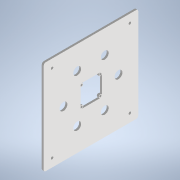
# Autodesk Inventor part: Plate
Saved by Autodesk Inventor 2022 (Build 260153000, 153)
## iProperties
Created: 2022-03-14
Part Number: Plate
Material: Generic
Document SubType Name: Modeling
Designer: ultra
Density: 1 g/cm^3
Appearance: Default
Author: ultra
Autodesk Inventor part; units mm, degrees
ref_plane "YZ Plane" through (0, 0, 0) normal (1, 0, 0) x (0, 1, 0)
ref_plane "XZ Plane" through (0, 0, 0) normal (0, 1, 0) x (-1, 0, 0)
ref_plane "XY Plane" through (0, 0, 0) normal (0, 0, 1) x (1, 0, 0)
sketch "Sketch1" plane through (0, 0, 0) normal (1, 0, 0) x (0, 1, 0)
  line L0 (-76.2, 76.2) -> (76.2, 76.2)
  line L1 (76.2, 76.2) -> (76.2, -76.2)
  line L2 (76.2, -76.2) -> (-76.2, -76.2)
  line L3 (-76.2, -76.2) -> (-76.2, 76.2)
  circle A0 centre (62.8611, 62.86) radius 2.032
  circle A1 centre (-62.8625, -62.8636) radius 2.032
  circle A2 centre (-0.0007, -88.9018) radius 2.032
  circle A3 centre (-62.8625, 62.86) radius 2.032
  circle A4 centre (88.8993, -0.0018) radius 2.032
  circle A5 centre (-88.9007, -0.0018) radius 2.032
  circle A6 centre (62.8611, -62.8636) radius 2.032
  circle A7 centre (-0.0007, 88.8982) radius 2.032
  circle A8 centre (-0.0007, -0.0018) radius 6.35
  dimension "d0" = 152.4
  dimension "d1" = 152.4
  dimension "d5" = 12.7
  constraints: 9 centre point, 8 end point, 2 parallel, 1 horizontal, 1 perpendicular
  measures "d0" distance of L1.end L2.end
  measures "d1" distance of L0.end L1.end
  measures "d5" diameter of A8
extrude "Extrusion2" add sketch "Sketch1" along normal blind 3.175 contours L0 L1 L2 L3 | A8
fillet "Fillet2" radius 3.175 4 edges at (1.5875, 76.2, 76.2) (1.5875, 76.2, -76.2) (1.5875, -76.2, 76.2) (1.5875, -76.2, -76.2)
sketch "Sketch2" plane through (3.175, 0, 0) normal (1, 0, 0) x (0, 0, -1)
  line L0 (-50.8, -50.8) -> (50.8, -50.8)
  line L1 (50.8, -50.8) -> (50.8, 50.8)
  line L2 (50.8, 50.8) -> (-50.8, 50.8)
  line L3 (-50.8, 50.8) -> (-50.8, -50.8)
  line L4 (-50.8, -50.8) -> (50.8, 50.8) construction
  line L5 (50.8, -50.8) -> (-50.8, 50.8) construction
  circle A0 centre (0, 0) radius 12.7
  line L6 (-12.7, 0) -> (-50.8, 38.1)
  line L7 (0, 12.7) -> (-38.1, 50.8)
  line L8 (-38.1, 50.8) -> (0, 12.7)
  line L9 (38.1, 50.8) -> (0, 12.7)
  line L10 (12.7, 0) -> (50.8, 38.1)
  line L11 (12.7, 0) -> (50.8, -38.1)
  line L12 (0, -12.7) -> (38.1, -50.8)
  line L13 (0, -12.7) -> (-38.1, -50.8)
  line L14 (-12.7, 0) -> (-50.8, -38.1)
  dimension "d9" = 101.6
  dimension "d10" = 101.6
  dimension "d11" = 25.4
  constraints: 30 end point, 10 point on line, 5 parallel, 4 point on circle, 2 midpoint, 2 perpendicular, 1 centre point, 1 coincident, 1 collinear, 1 horizontal
  measures "d9" distance of L2.end L1.end
  measures "d10" distance of L1.end L0.end
  measures "d11" diameter of A0
extrude "Extrusion3" [suppressed]
fillet "Fillet3" [suppressed]
sketch "Sketch3" plane through (3.175, 0, 0) normal (1, 0, 0) x (0, 0, -1)
  circle A0 centre (-22.225, -38.4948) radius 6.35
  circle A1 centre (-44.45, 0) radius 6.35
  circle A2 centre (22.225, -38.4948) radius 6.35
  circle A3 centre (-22.225, 38.4948) radius 6.35
  circle A4 centre (22.225, 38.4948) radius 6.35
  circle A5 centre (44.45, 0) radius 6.35
  point P0 (0, 0)
  constraints: 6 centre point
extrude "Extrusion4" cut sketch "Sketch3" against normal blind 25.4
sketch "Sketch4" plane through (3.175, 0, 0) normal (1, 0, 0) x (0, 0, -1)
  arc A0 (17.95, -14.8817) -> (14.6151, -17.9) centre (15.25, -15.25) ccw
  line L0 (17.95, -14.8817) -> (17.95, 14.8817)
  arc A1 (14.6151, 17.9) -> (17.95, 14.8817) centre (15.25, 15.25) ccw
  line L1 (14.6151, 17.9) -> (-14.6151, 17.9)
  arc A2 (-16.7532, 12.9771) -> (-14.6151, 17.9) centre (-15.25, 15.25) ccw
  arc A3 (-16.75, 12.9522) -> (-16.7532, 12.9771) centre (-16.85, 12.9522) ccw
  line L2 (-16.75, 12.9522) -> (-16.75, -12.9522)
  arc A4 (-16.7532, -12.9771) -> (-16.75, -12.9522) centre (-16.85, -12.9522) ccw
  arc A5 (-14.6151, -17.9) -> (-16.7532, -12.9771) centre (-15.25, -15.25) ccw
  line L3 (-14.6151, -17.9) -> (14.6151, -17.9)
  circle A6 centre (-11.1, -15.35) radius 0.6
  circle A7 centre (-11.1, -16.9) radius 0.6
  circle A8 centre (6.4427, -3.2254) radius 0.5
  line L4 (7.15, 15.83) -> (7.15, 17.17)
  arc A9 (7.07, 15.75) -> (7.15, 15.83) centre (7.07, 15.83) ccw
  line L5 (5.73, 15.75) -> (7.07, 15.75)
  arc A10 (5.65, 15.83) -> (5.73, 15.75) centre (5.73, 15.83) ccw
  line L6 (5.65, 17.17) -> (5.65, 15.83)
  arc A11 (5.73, 17.25) -> (5.65, 17.17) centre (5.73, 17.17) ccw
  line L7 (7.07, 17.25) -> (5.73, 17.25)
  arc A12 (7.15, 17.17) -> (7.07, 17.25) centre (7.07, 17.17) ccw
  line L8 (17.3, 4.83) -> (17.3, 6.17)
  arc A13 (17.22, 4.75) -> (17.3, 4.83) centre (17.22, 4.83) ccw
  line L9 (15.88, 4.75) -> (17.22, 4.75)
  arc A14 (15.8, 4.83) -> (15.88, 4.75) centre (15.88, 4.83) ccw
  line L10 (15.8, 6.17) -> (15.8, 4.83)
  arc A15 (15.88, 6.25) -> (15.8, 6.17) centre (15.88, 6.17) ccw
  line L11 (17.22, 6.25) -> (15.88, 6.25)
  arc A16 (17.3, 6.17) -> (17.22, 6.25) centre (17.22, 6.17) ccw
  line L12 (17.2, -10.52) -> (17.2, -9.18)
  arc A17 (17.12, -10.6) -> (17.2, -10.52) centre (17.12, -10.52) ccw
  line L13 (15.78, -10.6) -> (17.12, -10.6)
  arc A18 (15.7, -10.52) -> (15.78, -10.6) centre (15.78, -10.52) ccw
  line L14 (15.7, -9.18) -> (15.7, -10.52)
  arc A19 (15.78, -9.1) -> (15.7, -9.18) centre (15.78, -9.18) ccw
  line L15 (17.12, -9.1) -> (15.78, -9.1)
  arc A20 (17.2, -9.18) -> (17.12, -9.1) centre (17.12, -9.18) ccw
  line L16 (14.45, -7.97) -> (14.45, -6.63)
  arc A21 (14.37, -8.05) -> (14.45, -7.97) centre (14.37, -7.97) ccw
  line L17 (13.03, -8.05) -> (14.37, -8.05)
  arc A22 (12.95, -7.97) -> (13.03, -8.05) centre (13.03, -7.97) ccw
  line L18 (12.95, -6.63) -> (12.95, -7.97)
  arc A23 (13.03, -6.55) -> (12.95, -6.63) centre (13.03, -6.63) ccw
  line L19 (14.37, -6.55) -> (13.03, -6.55)
  arc A24 (14.45, -6.63) -> (14.37, -6.55) centre (14.37, -6.63) ccw
  line L20 (11.7, -11.52) -> (11.7, -10.18)
  arc A25 (11.62, -11.6) -> (11.7, -11.52) centre (11.62, -11.52) ccw
  line L21 (10.28, -11.6) -> (11.62, -11.6)
  arc A26 (10.2, -11.52) -> (10.28, -11.6) centre (10.28, -11.52) ccw
  line L22 (10.2, -10.18) -> (10.2, -11.52)
  arc A27 (10.28, -10.1) -> (10.2, -10.18) centre (10.28, -10.18) ccw
  line L23 (11.62, -10.1) -> (10.28, -10.1)
  arc A28 (11.7, -10.18) -> (11.62, -10.1) centre (11.62, -10.18) ccw
  circle A29 centre (6.25, -16.55) radius 0.75
  circle A30 centre (-12.95, -3.7) radius 0.6
  circle A31 centre (-12.95, -2.2) radius 0.6
  circle A32 centre (-12.95, -0.7) radius 0.6
  circle A33 centre (-15, -2.55) radius 0.5
  line L24 (9.55, -17.22) -> (9.55, -15.88)
  arc A34 (9.47, -17.3) -> (9.55, -17.22) centre (9.47, -17.22) ccw
  line L25 (8.13, -17.3) -> (9.47, -17.3)
  arc A35 (8.05, -17.22) -> (8.13, -17.3) centre (8.13, -17.22) ccw
  line L26 (8.05, -15.88) -> (8.05, -17.22)
  arc A36 (8.13, -15.8) -> (8.05, -15.88) centre (8.13, -15.88) ccw
  line L27 (9.47, -15.8) -> (8.13, -15.8)
  arc A37 (9.55, -15.88) -> (9.47, -15.8) centre (9.47, -15.88) ccw
  line L28 (7.15, 13.11) -> (7.15, 14.45)
  arc A38 (7.07, 13.03) -> (7.15, 13.11) centre (7.07, 13.11) ccw
  line L29 (5.73, 13.03) -> (7.07, 13.03)
  arc A39 (5.65, 13.11) -> (5.73, 13.03) centre (5.73, 13.11) ccw
  line L30 (5.65, 14.45) -> (5.65, 13.11)
  arc A40 (5.73, 14.53) -> (5.65, 14.45) centre (5.73, 14.45) ccw
  line L31 (7.07, 14.53) -> (5.73, 14.53)
  arc A41 (7.15, 14.45) -> (7.07, 14.53) centre (7.07, 14.45) ccw
  line L32 (5.6461, -4.7651) -> (6.9807, -4.7651)
  arc A42 (5.5661, -4.6851) -> (5.6461, -4.7651) centre (5.6461, -4.6851) ccw
  line L33 (5.5661, -4.143) -> (5.5661, -4.6851)
  arc A43 (5.6461, -4.063) -> (5.5661, -4.143) centre (5.6461, -4.143) ccw
  line L34 (6.9807, -4.063) -> (5.6461, -4.063)
  arc A44 (7.0607, -4.143) -> (6.9807, -4.063) centre (6.9807, -4.143) ccw
  line L35 (7.0607, -4.6851) -> (7.0607, -4.143)
  arc A45 (6.9807, -4.7651) -> (7.0607, -4.6851) centre (6.9807, -4.6851) ccw
  line L36 (5.7559, -12.4971) -> (7.4659, -12.4971)
  arc A46 (5.6759, -12.4171) -> (5.7559, -12.4971) centre (5.7559, -12.4171) ccw
  line L37 (5.6759, -11.4299) -> (5.6759, -12.4171)
  arc A47 (5.7559, -11.3499) -> (5.6759, -11.4299) centre (5.7559, -11.4299) ccw
  line L38 (7.4659, -11.3499) -> (5.7559, -11.3499)
  arc A48 (7.5459, -11.4299) -> (7.4659, -11.3499) centre (7.4659, -11.4299) ccw
  line L39 (7.5459, -12.4171) -> (7.5459, -11.4299)
  arc A49 (7.4659, -12.4971) -> (7.5459, -12.4171) centre (7.4659, -12.4171) ccw
  line L40 (-3.7607, -13.1472) -> (-6.2454, -13.1472)
  arc A50 (-3.6107, -13.2972) -> (-3.7607, -13.1472) centre (-3.7607, -13.2972) ccw
  line L41 (-3.6107, -13.9345) -> (-3.6107, -13.2972)
  arc A51 (-3.7607, -14.0845) -> (-3.6107, -13.9345) centre (-3.7607, -13.9345) ccw
  line L42 (-6.2454, -14.0845) -> (-3.7607, -14.0845)
  arc A52 (-6.3954, -13.9345) -> (-6.2454, -14.0845) centre (-6.2454, -13.9345) ccw
  line L43 (-6.3954, -13.2972) -> (-6.3954, -13.9345)
  arc A53 (-6.2454, -13.1472) -> (-6.3954, -13.2972) centre (-6.2454, -13.2972) ccw
  line L44 (-8.6796, 6.7587) -> (-7.8361, 6.7587)
  arc A54 (-8.7596, 6.8387) -> (-8.6796, 6.7587) centre (-8.6796, 6.8387) ccw
  line L45 (-8.7596, 7.1597) -> (-8.7596, 6.8387)
  arc A55 (-8.6796, 7.2397) -> (-8.7596, 7.1597) centre (-8.6796, 7.1597) ccw
  line L46 (-7.8361, 7.2397) -> (-8.6796, 7.2397)
  arc A56 (-7.7561, 7.1597) -> (-7.8361, 7.2397) centre (-7.8361, 7.1597) ccw
  line L47 (-7.7561, 6.8387) -> (-7.7561, 7.1597)
  arc A57 (-7.8361, 6.7587) -> (-7.7561, 6.8387) centre (-7.8361, 6.8387) ccw
  line L48 (-8.7273, 6.0564) -> (-8.7273, 5.7353)
  arc A58 (-8.6473, 6.1364) -> (-8.7273, 6.0564) centre (-8.6473, 6.0564) ccw
  line L49 (-7.8039, 6.1364) -> (-8.6473, 6.1364)
  arc A59 (-7.7239, 6.0564) -> (-7.8039, 6.1364) centre (-7.8039, 6.0564) ccw
  line L50 (-7.7239, 5.7353) -> (-7.7239, 6.0564)
  arc A60 (-7.8039, 5.6553) -> (-7.7239, 5.7353) centre (-7.8039, 5.7353) ccw
  line L51 (-8.6473, 5.6553) -> (-7.8039, 5.6553)
  arc A61 (-8.7273, 5.7353) -> (-8.6473, 5.6553) centre (-8.6473, 5.7353) ccw
  line L52 (-2.4248, 3.855) -> (-2.4248, 3.5921)
  arc A62 (-2.3448, 3.935) -> (-2.4248, 3.855) centre (-2.3448, 3.855) ccw
  line L53 (-1.6366, 3.935) -> (-2.3448, 3.935)
  arc A63 (-1.5566, 3.855) -> (-1.6366, 3.935) centre (-1.6366, 3.855) ccw
  line L54 (-1.5566, 3.5921) -> (-1.5566, 3.855)
  arc A64 (-1.6366, 3.5121) -> (-1.5566, 3.5921) centre (-1.6366, 3.5921) ccw
  line L55 (-2.3448, 3.5121) -> (-1.6366, 3.5121)
  arc A65 (-2.4248, 3.5921) -> (-2.3448, 3.5121) centre (-2.3448, 3.5921) ccw
  line L56 (-2.1101, 10.6062) -> (-2.1101, 10.3433)
  arc A66 (-2.0301, 10.6862) -> (-2.1101, 10.6062) centre (-2.0301, 10.6062) ccw
  line L57 (-1.3218, 10.6862) -> (-2.0301, 10.6862)
  arc A67 (-1.2418, 10.6062) -> (-1.3218, 10.6862) centre (-1.3218, 10.6062) ccw
  line L58 (-1.2418, 10.3433) -> (-1.2418, 10.6062)
  arc A68 (-1.3218, 10.2633) -> (-1.2418, 10.3433) centre (-1.3218, 10.3433) ccw
  line L59 (-2.0301, 10.2633) -> (-1.3218, 10.2633)
  arc A69 (-2.1101, 10.3433) -> (-2.0301, 10.2633) centre (-2.0301, 10.3433) ccw
  line L60 (4.251, 0.1966) -> (4.251, -0.0664)
  arc A70 (4.331, 0.2766) -> (4.251, 0.1966) centre (4.331, 0.1966) ccw
  line L61 (5.0392, 0.2766) -> (4.331, 0.2766)
  arc A71 (5.1192, 0.1966) -> (5.0392, 0.2766) centre (5.0392, 0.1966) ccw
  line L62 (5.1192, -0.0664) -> (5.1192, 0.1966)
  arc A72 (5.0392, -0.1464) -> (5.1192, -0.0664) centre (5.0392, -0.0664) ccw
  line L63 (4.331, -0.1464) -> (5.0392, -0.1464)
  arc A73 (4.251, -0.0664) -> (4.331, -0.1464) centre (4.331, -0.0664) ccw
  line L64 (4.251, -2.0073) -> (4.251, -2.2703)
  arc A74 (4.331, -1.9273) -> (4.251, -2.0073) centre (4.331, -2.0073) ccw
  line L65 (5.0392, -1.9273) -> (4.331, -1.9273)
  arc A75 (5.1192, -2.0073) -> (5.0392, -1.9273) centre (5.0392, -2.0073) ccw
  line L66 (5.1192, -2.2703) -> (5.1192, -2.0073)
  arc A76 (5.0392, -2.3503) -> (5.1192, -2.2703) centre (5.0392, -2.2703) ccw
  line L67 (4.331, -2.3503) -> (5.0392, -2.3503)
  arc A77 (4.251, -2.2703) -> (4.331, -2.3503) centre (4.331, -2.2703) ccw
  line L68 (5.5661, -5.3938) -> (5.5661, -5.6568)
  arc A78 (5.6461, -5.3138) -> (5.5661, -5.3938) centre (5.6461, -5.3938) ccw
  line L69 (6.3543, -5.3138) -> (5.6461, -5.3138)
  arc A79 (6.4343, -5.3938) -> (6.3543, -5.3138) centre (6.3543, -5.3938) ccw
  line L70 (6.4343, -5.6568) -> (6.4343, -5.3938)
  arc A80 (6.3543, -5.7368) -> (6.4343, -5.6568) centre (6.3543, -5.6568) ccw
  line L71 (5.6461, -5.7368) -> (6.3543, -5.7368)
  arc A81 (5.5661, -5.6568) -> (5.6461, -5.7368) centre (5.6461, -5.6568) ccw
  line L72 (5.6014, -10.4773) -> (5.6014, -10.7403)
  arc A82 (5.6814, -10.3973) -> (5.6014, -10.4773) centre (5.6814, -10.4773) ccw
  line L73 (6.3896, -10.3973) -> (5.6814, -10.3973)
  arc A83 (6.4696, -10.4773) -> (6.3896, -10.3973) centre (6.3896, -10.4773) ccw
  line L74 (6.4696, -10.7403) -> (6.4696, -10.4773)
  arc A84 (6.3896, -10.8203) -> (6.4696, -10.7403) centre (6.3896, -10.7403) ccw
  line L75 (5.6814, -10.8203) -> (6.3896, -10.8203)
  arc A85 (5.6014, -10.7403) -> (5.6814, -10.8203) centre (5.6814, -10.7403) ccw
  line L76 (-2.5133, -12.7708) -> (-2.5133, -13.0338)
  arc A86 (-2.4333, -12.6908) -> (-2.5133, -12.7708) centre (-2.4333, -12.7708) ccw
  line L77 (-1.7251, -12.6908) -> (-2.4333, -12.6908)
  arc A87 (-1.6451, -12.7708) -> (-1.7251, -12.6908) centre (-1.7251, -12.7708) ccw
  line L78 (-1.6451, -13.0338) -> (-1.6451, -12.7708)
  arc A88 (-1.7251, -13.1138) -> (-1.6451, -13.0338) centre (-1.7251, -13.0338) ccw
  line L79 (-2.4333, -13.1138) -> (-1.7251, -13.1138)
  arc A89 (-2.5133, -13.0338) -> (-2.4333, -13.1138) centre (-2.4333, -13.0338) ccw
  line L80 (-2.5327, -13.863) -> (-2.5327, -14.1668)
  arc A90 (-2.4527, -13.783) -> (-2.5327, -13.863) centre (-2.4527, -13.863) ccw
  line L81 (-1.6863, -13.783) -> (-2.4527, -13.783)
  arc A91 (-1.6063, -13.863) -> (-1.6863, -13.783) centre (-1.6863, -13.863) ccw
  line L82 (-1.6063, -14.1668) -> (-1.6063, -13.863)
  arc A92 (-1.6863, -14.2468) -> (-1.6063, -14.1668) centre (-1.6863, -14.1668) ccw
  line L83 (-2.4527, -14.2468) -> (-1.6863, -14.2468)
  arc A93 (-2.5327, -14.1668) -> (-2.4527, -14.2468) centre (-2.4527, -14.1668) ccw
  line L84 (-4.2466, 7.147) -> (-3.9765, 7.147)
  arc A94 (-4.3266, 7.227) -> (-4.2466, 7.147) centre (-4.2466, 7.227) ccw
  line L85 (-4.3266, 7.9294) -> (-4.3266, 7.227)
  arc A95 (-4.2466, 8.0094) -> (-4.3266, 7.9294) centre (-4.2466, 7.9294) ccw
  line L86 (-3.9765, 8.0094) -> (-4.2466, 8.0094)
  arc A96 (-3.8965, 7.9294) -> (-3.9765, 8.0094) centre (-3.9765, 7.9294) ccw
  line L87 (-3.8965, 7.227) -> (-3.8965, 7.9294)
  arc A97 (-3.9765, 7.147) -> (-3.8965, 7.227) centre (-3.9765, 7.227) ccw
  line L88 (-4.3762, 4.795) -> (-4.3762, 4.0926)
  arc A98 (-4.2962, 4.875) -> (-4.3762, 4.795) centre (-4.2962, 4.795) ccw
  line L89 (-4.0261, 4.875) -> (-4.2962, 4.875)
  arc A99 (-3.9461, 4.795) -> (-4.0261, 4.875) centre (-4.0261, 4.795) ccw
  line L90 (-3.9461, 4.0926) -> (-3.9461, 4.795)
  arc A100 (-4.0261, 4.0126) -> (-3.9461, 4.0926) centre (-4.0261, 4.0926) ccw
  line L91 (-4.2962, 4.0126) -> (-4.0261, 4.0126)
  arc A101 (-4.3762, 4.0926) -> (-4.2962, 4.0126) centre (-4.2962, 4.0926) ccw
  line L92 (-7.8593, 3.5305) -> (-7.8593, 2.8281)
  arc A102 (-7.7793, 3.6105) -> (-7.8593, 3.5305) centre (-7.7793, 3.5305) ccw
  line L93 (-7.5091, 3.6105) -> (-7.7793, 3.6105)
  arc A103 (-7.4291, 3.5305) -> (-7.5091, 3.6105) centre (-7.5091, 3.5305) ccw
  line L94 (-7.4291, 2.8281) -> (-7.4291, 3.5305)
  arc A104 (-7.5091, 2.7481) -> (-7.4291, 2.8281) centre (-7.5091, 2.8281) ccw
  line L95 (-7.7793, 2.7481) -> (-7.5091, 2.7481)
  arc A105 (-7.8593, 2.8281) -> (-7.7793, 2.7481) centre (-7.7793, 2.8281) ccw
  line L96 (8.2438, -6.8732) -> (8.2438, -7.5756)
  arc A106 (8.3238, -6.7932) -> (8.2438, -6.8732) centre (8.3238, -6.8732) ccw
  line L97 (8.594, -6.7932) -> (8.3238, -6.7932)
  arc A107 (8.674, -6.8732) -> (8.594, -6.7932) centre (8.594, -6.8732) ccw
  line L98 (8.674, -7.5756) -> (8.674, -6.8732)
  arc A108 (8.594, -7.6556) -> (8.674, -7.5756) centre (8.594, -7.5756) ccw
  line L99 (8.3238, -7.6556) -> (8.594, -7.6556)
  arc A109 (8.2438, -7.5756) -> (8.3238, -7.6556) centre (8.3238, -7.5756) ccw
  line L100 (4.0983, -7.1851) -> (4.0983, -7.8875)
  arc A110 (4.1783, -7.1051) -> (4.0983, -7.1851) centre (4.1783, -7.1851) ccw
  line L101 (4.4484, -7.1051) -> (4.1783, -7.1051)
  arc A111 (4.5284, -7.1851) -> (4.4484, -7.1051) centre (4.4484, -7.1851) ccw
  line L102 (4.5284, -7.8875) -> (4.5284, -7.1851)
  arc A112 (4.4484, -7.9675) -> (4.5284, -7.8875) centre (4.4484, -7.8875) ccw
  line L103 (4.1783, -7.9675) -> (4.4484, -7.9675)
  arc A113 (4.0983, -7.8875) -> (4.1783, -7.9675) centre (4.1783, -7.8875) ccw
  line L104 (1.7294, -13.1227) -> (1.7294, -13.8251)
  arc A114 (1.8094, -13.0427) -> (1.7294, -13.1227) centre (1.8094, -13.1227) ccw
  line L105 (2.0795, -13.0427) -> (1.8094, -13.0427)
  arc A115 (2.1595, -13.1227) -> (2.0795, -13.0427) centre (2.0795, -13.1227) ccw
  line L106 (2.1595, -13.8251) -> (2.1595, -13.1227)
  arc A116 (2.0795, -13.9051) -> (2.1595, -13.8251) centre (2.0795, -13.8251) ccw
  line L107 (1.8094, -13.9051) -> (2.0795, -13.9051)
  arc A117 (1.7294, -13.8251) -> (1.8094, -13.9051) centre (1.8094, -13.8251) ccw
  line L108 (0.6373, -13.1227) -> (0.6373, -13.8251)
  arc A118 (0.7173, -13.0427) -> (0.6373, -13.1227) centre (0.7173, -13.1227) ccw
  line L109 (0.9875, -13.0427) -> (0.7173, -13.0427)
  arc A119 (1.0675, -13.1227) -> (0.9875, -13.0427) centre (0.9875, -13.1227) ccw
  line L110 (1.0675, -13.8251) -> (1.0675, -13.1227)
  arc A120 (0.9875, -13.9051) -> (1.0675, -13.8251) centre (0.9875, -13.8251) ccw
  line L111 (0.7173, -13.9051) -> (0.9875, -13.9051)
  arc A121 (0.6373, -13.8251) -> (0.7173, -13.9051) centre (0.7173, -13.8251) ccw
  line L112 (-0.5491, -13.0325) -> (-0.5491, -13.8891)
  arc A122 (-0.4691, -12.9525) -> (-0.5491, -13.0325) centre (-0.4691, -13.0325) ccw
  line L113 (-0.0298, -12.9525) -> (-0.4691, -12.9525)
  arc A123 (0.0502, -13.0325) -> (-0.0298, -12.9525) centre (-0.0298, -13.0325) ccw
  line L114 (0.0502, -13.8891) -> (0.0502, -13.0325)
  arc A124 (-0.0298, -13.9691) -> (0.0502, -13.8891) centre (-0.0298, -13.8891) ccw
  line L115 (-0.4691, -13.9691) -> (-0.0298, -13.9691)
  arc A125 (-0.5491, -13.8891) -> (-0.4691, -13.9691) centre (-0.4691, -13.8891) ccw
  line L116 (-7.6347, -13.1227) -> (-7.6347, -13.8251)
  arc A126 (-7.5547, -13.0427) -> (-7.6347, -13.1227) centre (-7.5547, -13.1227) ccw
  line L117 (-7.2846, -13.0427) -> (-7.5547, -13.0427)
  arc A127 (-7.2046, -13.1227) -> (-7.2846, -13.0427) centre (-7.2846, -13.1227) ccw
  line L118 (-7.2046, -13.8251) -> (-7.2046, -13.1227)
  arc A128 (-7.2846, -13.9051) -> (-7.2046, -13.8251) centre (-7.2846, -13.8251) ccw
  line L119 (-7.5547, -13.9051) -> (-7.2846, -13.9051)
  arc A129 (-7.6347, -13.8251) -> (-7.5547, -13.9051) centre (-7.5547, -13.8251) ccw
  line L120 (-11.5137, -7.8762) -> (-11.5137, -8.5786)
  arc A130 (-11.4337, -7.7962) -> (-11.5137, -7.8762) centre (-11.4337, -7.8762) ccw
  line L121 (-11.1636, -7.7962) -> (-11.4337, -7.7962)
  arc A131 (-11.0836, -7.8762) -> (-11.1636, -7.7962) centre (-11.1636, -7.8762) ccw
  line L122 (-11.0836, -8.5786) -> (-11.0836, -7.8762)
  arc A132 (-11.1636, -8.6586) -> (-11.0836, -8.5786) centre (-11.1636, -8.5786) ccw
  line L123 (-11.4337, -8.6586) -> (-11.1636, -8.6586)
  arc A133 (-11.5137, -8.5786) -> (-11.4337, -8.6586) centre (-11.4337, -8.5786) ccw
  line L124 (-11.5137, -5.7855) -> (-11.5137, -6.4879)
  arc A134 (-11.4337, -5.7055) -> (-11.5137, -5.7855) centre (-11.4337, -5.7855) ccw
  line L125 (-11.1636, -5.7055) -> (-11.4337, -5.7055)
  arc A135 (-11.0836, -5.7855) -> (-11.1636, -5.7055) centre (-11.1636, -5.7855) ccw
  line L126 (-11.0836, -6.4879) -> (-11.0836, -5.7855)
  arc A136 (-11.1636, -6.5679) -> (-11.0836, -6.4879) centre (-11.1636, -6.4879) ccw
  line L127 (-11.4337, -6.5679) -> (-11.1636, -6.5679)
  arc A137 (-11.5137, -6.4879) -> (-11.4337, -6.5679) centre (-11.4337, -6.4879) ccw
  line L128 (-6.8045, 2.6819) -> (-6.3852, 2.6819)
  arc A138 (-6.8845, 2.7619) -> (-6.8045, 2.6819) centre (-6.8045, 2.7619) ccw
  line L129 (-6.8845, 3.604) -> (-6.8845, 2.7619)
  arc A139 (-6.8045, 3.684) -> (-6.8845, 3.604) centre (-6.8045, 3.604) ccw
  line L130 (-6.3852, 3.684) -> (-6.8045, 3.684)
  arc A140 (-6.3052, 3.604) -> (-6.3852, 3.684) centre (-6.3852, 3.604) ccw
  line L131 (-6.3052, 2.7619) -> (-6.3052, 3.604)
  arc A141 (-6.3852, 2.6819) -> (-6.3052, 2.7619) centre (-6.3852, 2.7619) ccw
  line L132 (4.2459, -1.3202) -> (5.1267, -1.3202)
  arc A142 (4.1659, -1.2402) -> (4.2459, -1.3202) centre (4.2459, -1.2402) ccw
  line L133 (4.1659, -0.8183) -> (4.1659, -1.2402)
  arc A143 (4.2459, -0.7383) -> (4.1659, -0.8183) centre (4.2459, -0.8183) ccw
  line L134 (5.1267, -0.7383) -> (4.2459, -0.7383)
  arc A144 (5.2067, -0.8183) -> (5.1267, -0.7383) centre (5.1267, -0.8183) ccw
  line L135 (5.2067, -1.2402) -> (5.2067, -0.8183)
  arc A145 (5.1267, -1.3202) -> (5.2067, -1.2402) centre (5.1267, -1.2402) ccw
  line L136 (8.5655, 12.3987) -> (9.3164, 12.3987)
  arc A146 (8.4855, 12.4787) -> (8.5655, 12.3987) centre (8.5655, 12.4787) ccw
  line L137 (8.4855, 13.8248) -> (8.4855, 12.4787)
  arc A147 (8.5655, 13.9048) -> (8.4855, 13.8248) centre (8.5655, 13.8248) ccw
  line L138 (9.3164, 13.9048) -> (8.5655, 13.9048)
  arc A148 (9.3964, 13.8248) -> (9.3164, 13.9048) centre (9.3164, 13.8248) ccw
  line L139 (9.3964, 12.4787) -> (9.3964, 13.8248)
  arc A149 (9.3164, 12.3987) -> (9.3964, 12.4787) centre (9.3164, 12.4787) ccw
  line L140 (8.5655, 15.1054) -> (9.234, 15.1054)
  arc A150 (8.4855, 15.1854) -> (8.5655, 15.1054) centre (8.5655, 15.1854) ccw
  line L141 (8.4855, 16.6154) -> (8.4855, 15.1854)
  arc A151 (8.5655, 16.6954) -> (8.4855, 16.6154) centre (8.5655, 16.6154) ccw
  line L142 (9.234, 16.6954) -> (8.5655, 16.6954)
  arc A152 (9.314, 16.6154) -> (9.234, 16.6954) centre (9.234, 16.6154) ccw
  line L143 (9.314, 15.1854) -> (9.314, 16.6154)
  arc A153 (9.234, 15.1054) -> (9.314, 15.1854) centre (9.234, 15.1854) ccw
  line L144 (3.1491, 10.119) -> (3.4442, 10.119)
  arc A154 (3.0691, 10.199) -> (3.1491, 10.119) centre (3.1491, 10.199) ccw
  line L145 (3.0691, 10.9694) -> (3.0691, 10.199)
  arc A155 (3.1491, 11.0494) -> (3.0691, 10.9694) centre (3.1491, 10.9694) ccw
  line L146 (3.4442, 11.0494) -> (3.1491, 11.0494)
  arc A156 (3.5242, 10.9694) -> (3.4442, 11.0494) centre (3.4442, 10.9694) ccw
  line L147 (3.5242, 10.199) -> (3.5242, 10.9694)
  arc A157 (3.4442, 10.119) -> (3.5242, 10.199) centre (3.4442, 10.199) ccw
  line L148 (4.1659, 10.941) -> (4.1659, 10.1706)
  arc A158 (4.2459, 11.021) -> (4.1659, 10.941) centre (4.2459, 10.941) ccw
  line L149 (4.5409, 11.021) -> (4.2459, 11.021)
  arc A159 (4.6209, 10.941) -> (4.5409, 11.021) centre (4.5409, 10.941) ccw
  line L150 (4.6209, 10.1706) -> (4.6209, 10.941)
  arc A160 (4.5409, 10.0906) -> (4.6209, 10.1706) centre (4.5409, 10.1706) ccw
  line L151 (4.2459, 10.0906) -> (4.5409, 10.0906)
  arc A161 (4.1659, 10.1706) -> (4.2459, 10.0906) centre (4.2459, 10.1706) ccw
  line L152 (5.2631, 10.941) -> (5.2631, 10.1706)
  arc A162 (5.3431, 11.021) -> (5.2631, 10.941) centre (5.3431, 10.941) ccw
  line L153 (5.6381, 11.021) -> (5.3431, 11.021)
  arc A163 (5.7181, 10.941) -> (5.6381, 11.021) centre (5.6381, 10.941) ccw
  line L154 (5.7181, 10.1706) -> (5.7181, 10.941)
  arc A164 (5.6381, 10.0906) -> (5.7181, 10.1706) centre (5.6381, 10.1706) ccw
  line L155 (5.3431, 10.0906) -> (5.6381, 10.0906)
  arc A165 (5.2631, 10.1706) -> (5.3431, 10.0906) centre (5.3431, 10.1706) ccw
  line L156 (6.7177, 10.941) -> (6.7177, 10.1706)
  arc A166 (6.7977, 11.021) -> (6.7177, 10.941) centre (6.7977, 10.941) ccw
  line L157 (7.0927, 11.021) -> (6.7977, 11.021)
  arc A167 (7.1727, 10.941) -> (7.0927, 11.021) centre (7.0927, 10.941) ccw
  line L158 (7.1727, 10.1706) -> (7.1727, 10.941)
  arc A168 (7.0927, 10.0906) -> (7.1727, 10.1706) centre (7.0927, 10.1706) ccw
  line L159 (6.7977, 10.0906) -> (7.0927, 10.0906)
  arc A169 (6.7177, 10.1706) -> (6.7977, 10.0906) centre (6.7977, 10.1706) ccw
  line L160 (7.7678, 10.895) -> (7.7678, 10.1246)
  arc A170 (7.8478, 10.975) -> (7.7678, 10.895) centre (7.8478, 10.895) ccw
  line L161 (8.1429, 10.975) -> (7.8478, 10.975)
  arc A171 (8.2229, 10.895) -> (8.1429, 10.975) centre (8.1429, 10.895) ccw
  line L162 (8.2229, 10.1246) -> (8.2229, 10.895)
  arc A172 (8.1429, 10.0446) -> (8.2229, 10.1246) centre (8.1429, 10.1246) ccw
  line L163 (7.8478, 10.0446) -> (8.1429, 10.0446)
  arc A173 (7.7678, 10.1246) -> (7.8478, 10.0446) centre (7.8478, 10.1246) ccw
  line L164 (4.1659, 8.6981) -> (4.1659, 7.9277)
  arc A174 (4.2459, 8.7781) -> (4.1659, 8.6981) centre (4.2459, 8.6981) ccw
  line L165 (4.5409, 8.7781) -> (4.2459, 8.7781)
  arc A175 (4.6209, 8.6981) -> (4.5409, 8.7781) centre (4.5409, 8.6981) ccw
  line L166 (4.6209, 7.9277) -> (4.6209, 8.6981)
  arc A176 (4.5409, 7.8477) -> (4.6209, 7.9277) centre (4.5409, 7.9277) ccw
  line L167 (4.2459, 7.8477) -> (4.5409, 7.8477)
  arc A177 (4.1659, 7.9277) -> (4.2459, 7.8477) centre (4.2459, 7.9277) ccw
  line L168 (4.1422, 6.6231) -> (4.1422, 5.8527)
  arc A178 (4.2222, 6.7031) -> (4.1422, 6.6231) centre (4.2222, 6.6231) ccw
  line L169 (4.5172, 6.7031) -> (4.2222, 6.7031)
  arc A179 (4.5972, 6.6231) -> (4.5172, 6.7031) centre (4.5172, 6.6231) ccw
  line L170 (4.5972, 5.8527) -> (4.5972, 6.6231)
  arc A180 (4.5172, 5.7727) -> (4.5972, 5.8527) centre (4.5172, 5.8527) ccw
  line L171 (4.2222, 5.7727) -> (4.5172, 5.7727)
  arc A181 (4.1422, 5.8527) -> (4.2222, 5.7727) centre (4.2222, 5.8527) ccw
  line L172 (4.331, -14.4484) -> (5.6381, -14.4484)
  arc A182 (4.251, -14.3684) -> (4.331, -14.4484) centre (4.331, -14.3684) ccw
  line L173 (4.251, -13.7408) -> (4.251, -14.3684)
  arc A183 (4.331, -13.6608) -> (4.251, -13.7408) centre (4.331, -13.7408) ccw
  line L174 (5.6381, -13.6608) -> (4.331, -13.6608)
  arc A184 (5.7181, -13.7408) -> (5.6381, -13.6608) centre (5.6381, -13.7408) ccw
  line L175 (5.7181, -14.3684) -> (5.7181, -13.7408)
  arc A185 (5.6381, -14.4484) -> (5.7181, -14.3684) centre (5.6381, -14.3684) ccw
  line L176 (7.0497, -14.4484) -> (8.471, -14.4484)
  arc A186 (6.9697, -14.3684) -> (7.0497, -14.4484) centre (7.0497, -14.3684) ccw
  line L177 (6.9697, -13.7408) -> (6.9697, -14.3684)
  arc A187 (7.0497, -13.6608) -> (6.9697, -13.7408) centre (7.0497, -13.7408) ccw
  line L178 (8.471, -13.6608) -> (7.0497, -13.6608)
  arc A188 (8.551, -13.7408) -> (8.471, -13.6608) centre (8.471, -13.7408) ccw
  line L179 (8.551, -14.3684) -> (8.551, -13.7408)
  arc A189 (8.471, -14.4484) -> (8.551, -14.3684) centre (8.471, -14.3684) ccw
  line L180 (16.0437, 3.0276) -> (16.0437, 3.4967)
  line L181 (16.7651, 3.0276) -> (16.0437, 3.0276)
  arc A190 (16.9393, 2.8534) -> (16.7651, 3.0276) centre (16.7651, 2.8534) ccw
  line L182 (16.9393, 2.6792) -> (16.9393, 2.8534)
  arc A191 (16.7651, 2.505) -> (16.9393, 2.6792) centre (16.7651, 2.6792) ccw
  line L183 (16.0437, 2.505) -> (16.7651, 2.505)
  line L184 (16.0437, 1.7552) -> (16.0437, 2.505)
  line L185 (16.7651, 1.7552) -> (16.0437, 1.7552)
  arc A192 (16.9393, 1.581) -> (16.7651, 1.7552) centre (16.7651, 1.581) ccw
  line L186 (16.9393, 1.4068) -> (16.9393, 1.581)
  arc A193 (16.7651, 1.2326) -> (16.9393, 1.4068) centre (16.7651, 1.4068) ccw
  line L187 (16.0437, 1.2326) -> (16.7651, 1.2326)
  line L188 (16.0437, 0.4828) -> (16.0437, 1.2326)
  line L189 (16.7651, 0.4828) -> (16.0437, 0.4828)
  arc A194 (16.9393, 0.3086) -> (16.7651, 0.4828) centre (16.7651, 0.3086) ccw
  line L190 (16.9393, 0.1344) -> (16.9393, 0.3086)
  arc A195 (16.7651, -0.0398) -> (16.9393, 0.1344) centre (16.7651, 0.1344) ccw
  line L191 (16.0437, -0.0398) -> (16.7651, -0.0398)
  line L192 (16.0437, -0.7897) -> (16.0437, -0.0398)
  line L193 (16.7651, -0.7897) -> (16.0437, -0.7897)
  arc A196 (16.9393, -0.9638) -> (16.7651, -0.7897) centre (16.7651, -0.9638) ccw
  line L194 (16.9393, -1.138) -> (16.9393, -0.9638)
  arc A197 (16.7651, -1.3122) -> (16.9393, -1.138) centre (16.7651, -1.138) ccw
  line L195 (16.0437, -1.3122) -> (16.7651, -1.3122)
  line L196 (16.0437, -2.0621) -> (16.0437, -1.3122)
  line L197 (16.7651, -2.0621) -> (16.0437, -2.0621)
  arc A198 (16.9393, -2.2362) -> (16.7651, -2.0621) centre (16.7651, -2.2362) ccw
  line L198 (16.9393, -2.4104) -> (16.9393, -2.2362)
  arc A199 (16.7651, -2.5846) -> (16.9393, -2.4104) centre (16.7651, -2.4104) ccw
  line L199 (16.0437, -2.5846) -> (16.7651, -2.5846)
  line L200 (16.0437, -3.2742) -> (16.0437, -2.5846)
  line L201 (13.0463, -3.2742) -> (16.0437, -3.2742)
  line L202 (13.0463, -2.5846) -> (13.0463, -3.2742)
  line L203 (12.3249, -2.5846) -> (13.0463, -2.5846)
  arc A200 (12.1507, -2.4104) -> (12.3249, -2.5846) centre (12.3249, -2.4104) ccw
  line L204 (12.1507, -2.2362) -> (12.1507, -2.4104)
  arc A201 (12.3249, -2.0621) -> (12.1507, -2.2362) centre (12.3249, -2.2362) ccw
  line L205 (13.0463, -2.0621) -> (12.3249, -2.0621)
  line L206 (13.0463, -1.3122) -> (13.0463, -2.0621)
  line L207 (12.3249, -1.3122) -> (13.0463, -1.3122)
  arc A202 (12.1507, -1.138) -> (12.3249, -1.3122) centre (12.3249, -1.138) ccw
  line L208 (12.1507, -0.9638) -> (12.1507, -1.138)
  arc A203 (12.3249, -0.7897) -> (12.1507, -0.9638) centre (12.3249, -0.9638) ccw
  line L209 (13.0463, -0.7897) -> (12.3249, -0.7897)
  line L210 (13.0463, -0.0398) -> (13.0463, -0.7897)
  line L211 (12.3249, -0.0398) -> (13.0463, -0.0398)
  arc A204 (12.1507, 0.1344) -> (12.3249, -0.0398) centre (12.3249, 0.1344) ccw
  line L212 (12.1507, 0.3086) -> (12.1507, 0.1344)
  arc A205 (12.3249, 0.4828) -> (12.1507, 0.3086) centre (12.3249, 0.3086) ccw
  line L213 (13.0463, 0.4828) -> (12.3249, 0.4828)
  line L214 (13.0463, 1.2326) -> (13.0463, 0.4828)
  line L215 (12.3249, 1.2326) -> (13.0463, 1.2326)
  arc A206 (12.1507, 1.4068) -> (12.3249, 1.2326) centre (12.3249, 1.4068) ccw
  line L216 (12.1507, 1.581) -> (12.1507, 1.4068)
  arc A207 (12.3249, 1.7552) -> (12.1507, 1.581) centre (12.3249, 1.581) ccw
  line L217 (13.0463, 1.7552) -> (12.3249, 1.7552)
  line L218 (13.0463, 2.505) -> (13.0463, 1.7552)
  line L219 (12.3249, 2.505) -> (13.0463, 2.505)
  arc A208 (12.1507, 2.6792) -> (12.3249, 2.505) centre (12.3249, 2.6792) ccw
  line L220 (12.1507, 2.8534) -> (12.1507, 2.6792)
  arc A209 (12.3249, 3.0276) -> (12.1507, 2.8534) centre (12.3249, 2.8534) ccw
  line L221 (13.0463, 3.0276) -> (12.3249, 3.0276)
  line L222 (13.0463, 3.4967) -> (13.0463, 3.0276)
  line L223 (16.0437, 3.4967) -> (13.0463, 3.4967)
  line L224 (5.0276, -8.661) -> (7.7758, -8.661)
  arc A210 (4.9476, -8.581) -> (5.0276, -8.661) centre (5.0276, -8.581) ccw
  line L225 (4.9476, -7.1347) -> (4.9476, -8.581)
  arc A211 (5.0276, -7.0547) -> (4.9476, -7.1347) centre (5.0276, -7.1347) ccw
  line L226 (7.7758, -7.0547) -> (5.0276, -7.0547)
  arc A212 (7.8558, -7.1347) -> (7.7758, -7.0547) centre (7.7758, -7.1347) ccw
  line L227 (7.8558, -8.581) -> (7.8558, -7.1347)
  arc A213 (7.7758, -8.661) -> (7.8558, -8.581) centre (7.7758, -8.581) ccw
  line L228 (6.0886, 5.3054) -> (7.1066, 5.3054)
  arc A214 (6.0086, 5.3854) -> (6.0886, 5.3054) centre (6.0886, 5.3854) ccw
  line L229 (6.0086, 7.9827) -> (6.0086, 5.3854)
  arc A215 (6.0886, 8.0627) -> (6.0086, 7.9827) centre (6.0886, 7.9827) ccw
  line L230 (7.1066, 8.0627) -> (6.0886, 8.0627)
  arc A216 (7.1866, 7.9827) -> (7.1066, 8.0627) centre (7.1066, 7.9827) ccw
  line L231 (7.1866, 5.3854) -> (7.1866, 7.9827)
  arc A217 (7.1066, 5.3054) -> (7.1866, 5.3854) centre (7.1066, 5.3854) ccw
  line L232 (-8.4617, 7.7077) -> (-6.9198, 7.7077)
  arc A218 (-8.5417, 7.7877) -> (-8.4617, 7.7077) centre (-8.4617, 7.7877) ccw
  line L233 (-8.5417, 8.7477) -> (-8.5417, 7.7877)
  arc A219 (-8.4617, 8.8277) -> (-8.5417, 8.7477) centre (-8.4617, 8.7477) ccw
  line L234 (-6.9198, 8.8277) -> (-8.4617, 8.8277)
  arc A220 (-6.8398, 8.7477) -> (-6.9198, 8.8277) centre (-6.9198, 8.7477) ccw
  line L235 (-6.8398, 7.7877) -> (-6.8398, 8.7477)
  arc A221 (-6.9198, 7.7077) -> (-6.8398, 7.7877) centre (-6.9198, 7.7877) ccw
  line L236 (-8.518, 9.6348) -> (-6.9198, 9.6348)
  arc A222 (-8.598, 9.7148) -> (-8.518, 9.6348) centre (-8.518, 9.7148) ccw
  line L237 (-8.598, 10.7186) -> (-8.598, 9.7148)
  arc A223 (-8.518, 10.7986) -> (-8.598, 10.7186) centre (-8.518, 10.7186) ccw
  line L238 (-6.9198, 10.7986) -> (-8.518, 10.7986)
  arc A224 (-6.8398, 10.7186) -> (-6.9198, 10.7986) centre (-6.9198, 10.7186) ccw
  line L239 (-6.8398, 9.7148) -> (-6.8398, 10.7186)
  arc A225 (-6.9198, 9.6348) -> (-6.8398, 9.7148) centre (-6.9198, 9.7148) ccw
  line L240 (-2.7165, 5.1018) -> (1.1034, 5.1018)
  arc A226 (-2.7965, 5.1818) -> (-2.7165, 5.1018) centre (-2.7165, 5.1818) ccw
  line L241 (-2.7965, 9.0135) -> (-2.7965, 5.1818)
  arc A227 (-2.7165, 9.0935) -> (-2.7965, 9.0135) centre (-2.7165, 9.0135) ccw
  line L242 (1.1034, 9.0935) -> (-2.7165, 9.0935)
  arc A228 (1.1834, 9.0135) -> (1.1034, 9.0935) centre (1.1034, 9.0135) ccw
  line L243 (1.1834, 5.1818) -> (1.1834, 9.0135)
  arc A229 (1.1034, 5.1018) -> (1.1834, 5.1818) centre (1.1034, 5.1818) ccw
  circle A230 centre (3.7, -16.55) radius 0.75
  circle A231 centre (1.15, -16.55) radius 0.75
  circle A232 centre (-1.4, -16.55) radius 0.75
  circle A233 centre (-3.95, -16.55) radius 0.75
  circle A234 centre (-6.5, -16.55) radius 0.75
  circle A235 centre (-9.05, -16.55) radius 0.75
  circle A236 centre (3.9, 13.78) radius 0.75
  circle A237 centre (16.55, 8.05) radius 0.75
  circle A238 centre (16.45, -7.3) radius 0.75
  circle A239 centre (13.7, -9.85) radius 0.75
  circle A240 centre (10.95, -8.3) radius 0.75
  circle A241 centre (10.95, -5.75) radius 0.75
  circle A242 centre (-1.2, 16.5) radius 0.75
  circle A243 centre (-3.75, 16.5) radius 0.75
  circle A244 centre (-6.3, 16.5) radius 0.75
  circle A245 centre (1.35, 13.78) radius 0.75
  circle A246 centre (-1.2, 13.78) radius 0.75
  circle A247 centre (-3.75, 13.78) radius 0.75
  circle A248 centre (1.35, 16.5) radius 0.75
  circle A249 centre (3.9, 16.5) radius 0.75
  circle A250 centre (-6.3, 13.78) radius 0.75
  circle A251 centre (-11.4, -1.15) radius 0.6
  circle A252 centre (-11.4, -2.65) radius 0.6
  circle A253 centre (-11.4, -4.15) radius 0.6
  circle A254 centre (-11.1, -10.85) radius 0.6
  circle A255 centre (-11.1, -13.85) radius 0.6
  circle A256 centre (-11.1, -12.3) radius 0.65
  circle A257 centre (-5.7697, 6.8702) radius 0.5
  circle A258 centre (-6.6288, 5.896) radius 0.5
  circle A259 centre (15.25, -15.25) radius 2.725
  circle A260 centre (-15.25, -15.25) radius 2.725
  circle A261 centre (-15.25, 15.25) radius 2.725
  circle A262 centre (15.25, 15.25) radius 2.725
  circle A263 centre (15.25, -15.25) radius 1.75
  circle A264 centre (-15.25, -15.25) radius 1.75
  circle A265 centre (-15.25, 15.25) radius 1.75
  circle A266 centre (15.25, 15.25) radius 1.75
  point P0 (0, 0)
  point P1 (0, 0)
  point P2 (17.95, 14.8817)
  point P3 (14.6151, -17.9)
  dimension "d19" = 2.725
  dimension "d20" = 3.5
  dimension "d21" = 3.5
  dimension "d22" = 3.5
  dimension "d23" = 3.5
  constraints: 488 end point, 444 point on circle, 267 centre point, 8 coincident, 3 concentric
  measures "d19" radius of A0
  measures "d20" diameter of A263
  measures "d21" diameter of A264
  measures "d22" diameter of A265
  measures "d23" diameter of A266
extrude "Extrusion6" cut sketch "Sketch4" against normal blind 25.4 contours A263 | A264 | A265 | A266
body "Solid2"
